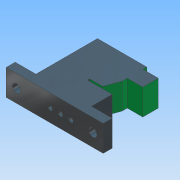
# Autodesk Inventor part: Ventil_Inside
Saved by Autodesk Inventor 2016 (Build 200138000, 138)
## iProperties
Created: 2011-05-25
Part Number: Ventil_Inside
Material: Thermoplastic Resin
Document SubType Name: Modeling
Designer: Neef
Mass: 7.93981 g
Surface Area: 28.866 cm^2
Volume: 6.20297 cm^3
Density: 1.28 g/cm^3
Appearance: Smooth - Medium Gray
Author: Neef
Autodesk Inventor part; units mm, degrees
ref_plane "YZ Plane" through (0, 0, 0) normal (1, 0, 0) x (0, 1, 0)
ref_plane "XZ Plane" through (0, 0, 0) normal (0, 1, 0) x (-1, 0, 0)
ref_plane "XY Plane" through (0, 0, 0) normal (0, 0, 1) x (1, 0, 0)
sketch "Skizze1" plane through (0, 0, 0) normal (0, 0, 1) x (1, 0, 0)
  line L0 (0, 0) -> (0, 3.5)
  line L1 (0, 3.5) -> (8, 3.5)
  line L2 (8, 3.5) -> (8, 27.3)
  line L3 (8, 27.3) -> (27, 27.3)
  line L4 (27, 27.3) -> (27, 25.795)
  line L5 (27, 25.795) -> (33, 25.795)
  line L6 (33, 25.795) -> (33, 19.795)
  line L7 (33, 19.795) -> (27, 19.795)
  line L8 (27, 19.795) -> (27, 17.795)
  line L9 (27, 17.795) -> (25, 12.3)
  line L10 (25, 12.3) -> (20, 12.3)
  line L11 (20, 12.3) -> (20, 11.5)
  line L12 (20, 11.5) -> (29.5, 11.5)
  line L13 (29.5, 11.5) -> (29.5, 3.5)
  line L14 (29.5, 3.5) -> (37.5, 3.5)
  line L15 (37.5, 3.5) -> (37.5, 0)
  line L16 (37.5, 0) -> (0, 0)
  line L17 (0, 32.76) -> (0, -5.46) projected
  line L18 (-7.5, 0) -> (45, 0) projected
  dimension "d0" = 27.3
  dimension "d1" = 3.5
  dimension "d2" = 37.5
  dimension "d3" = 8
  dimension "d4" = 19
  dimension "d5" = 6
  dimension "d6" = 6
  dimension "d7" = 15
  dimension "d8" = 11.5
  dimension "d9" = 21.5
  dimension "d10" = 12
  dimension "d11" = 17
  dimension "d12" = 2
  dimension "d13" = 70
  constraints: 34 end point, 12 parallel, 3 perpendicular, 2 point on line, 1 vertical
  measures "d0" distance between parallel lines of L3 L16
  measures "d1" distance of L0.start L0.end
  measures "d2" distance of L15.end L0.start
  measures "d3" distance of L0.end L1.end
  measures "d4" distance of L2.end L3.end
  measures "d5" distance of L4.end L5.end
  measures "d6" distance of L5.end L6.end
  measures "d7" distance between parallel lines of L3 L10
  measures "d8" distance between parallel lines of L16 L12
  measures "d9" distance between parallel lines of L2 L13
  measures "d10" distance between parallel lines of L11 L2
  measures "d11" distance from line of L2 L9.end
  measures "d12" distance of L7.end L8.end
  measures "d13" angle of L18 L9
extrude "Extrusion1" add sketch "Skizze1" along normal blind 10
sketch "Skizze2" plane through (0, 0, 0) normal (0, -1, 0) x (1, 0, 0)
  line L0 (37.5, 10) -> (0, 10) projected
  line L1 (37.5, 0) -> (37.5, 10) projected
  point P0 (25, 5)
  point P1 (17, 5)
  point P2 (21, 5)
  dimension "d16" = 16.5
  dimension "d17" = 4
  dimension "d18" = 4
  dimension "d19" = 5
  dimension "d20" = 5
  dimension "d21" = 5
  measures "d16" distance from line of L1 point (21, 5)
  measures "d17" distance of point (21, 5) point (25, 5)
  measures "d18" distance of point (21, 5) point (17, 5)
  measures "d19" distance from line of L0 point (17, 5)
  measures "d20" distance from line of L0 point (21, 5)
  measures "d21" distance from line of L0 point (25, 5)
hole "Bohrung1" at (25, 0, 5) at (17, 0, 5) at (21, 0, 5) direction (0, 1, 0) diameter 1.8 depth 3 tip angle 118
sketch "Skizze3" plane through (0, 0, 0) normal (0, -1, 0) x (1, 0, 0)
  circle A0 centre (21, 5) radius 0.9 projected
  line L0 (37.5, 10) -> (0, 10) projected
  point P0 (33.5, 5)
  point P1 (4, 5)
  dimension "d30" = 12.5
  dimension "d31" = 17
  dimension "d32" = 5
  dimension "d33" = 5
  measures "d30" distance of point (33.5, 5) A0.centre
  measures "d31" distance of point (4, 5) A0.centre
  measures "d32" distance from line of point (33.5, 5) L0
  measures "d33" distance from line of point (4, 5) L0
hole "Bohrung2" at (33.5, 0, 5) at (4, 0, 5) direction (0, 1, 0) diameter 3.2 depth 3.5 tip angle 118 clearance for "Inbusschraube DIN EN ISO 4762" size "M3" standard "DIN"
equation "\"d18\" = d17"
equation "\"d20\" = d19"
equation "\"d21\" = d19"
